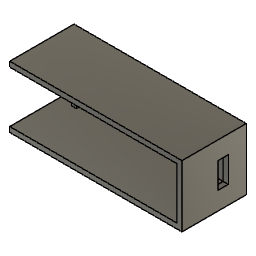
usb-bracket v4 (Autodesk Fusion 360 design; units mm, degrees)
Autodesk Fusion 360 part; units mm, degrees
sketch "Sketch1" plane through (0, 0, 0) normal (0, 1, 0) x (1, 0, 0)
  line L0 (0, 0) -> (-58, 0)
  line L1 (-58, 0) -> (-58, -20)
  line L2 (-58, -20) -> (0, -20)
  line L3 (0, -20) -> (0, 0)
  constraint horizontal L0
  constraint vertical L1
  constraint horizontal L2
  constraint vertical L3
  constraint coincident L0.start L3.end
extrude "Extrude1" add sketch "Sketch1" against normal blind 2
sketch "Sketch2" plane through (0, 0, 0) normal (0, 1, 0) x (1, 0, 0)
  line L0 (-60, -22) -> (2, -22)
  line L1 (2, -22) -> (2, -20)
  line L2 (2, -20) -> (-60, -20)
  line L3 (-60, -20) -> (-60, -22)
  constraint horizontal L0
  constraint vertical L1
  constraint horizontal L2
  constraint vertical L3
extrude "Extrude2" add sketch "Sketch2" against normal blind 7
sketch "Sketch3" plane through (0, 0, 0) normal (0, 1, 0) x (1, 0, 0)
  line L0 (-60, 0) -> (2, 0)
  line L1 (2, 0) -> (2, 2)
  line L2 (2, 2) -> (-60, 2)
  line L3 (-60, 2) -> (-60, 0)
  constraint horizontal L0
  constraint vertical L1
  constraint horizontal L2
  constraint vertical L3
extrude "Extrude3" add sketch "Sketch3" against normal blind 7
sketch "Sketch4" plane through (0, 0, 0) normal (0, 1, 0) x (1, 0, 0)
  line L0 (0, -20) -> (2, -20)
  line L1 (2, -20) -> (2, 0)
  line L2 (2, 0) -> (0, 0)
  line L3 (0, 0) -> (0, -20)
  constraint horizontal L0
  constraint vertical L1
  constraint horizontal L2
  constraint vertical L3
extrude "Extrude4" add sketch "Sketch4" against normal blind 7
sketch "Sketch5" plane through (0, 0, 0) normal (0, 1, 0) x (1, 0, 0)
  line L0 (-42, -20) -> (-37, -20)
  line L1 (-37, -20) -> (-37, 0)
  line L2 (-37, 0) -> (-42, 0)
  line L3 (-42, 0) -> (-42, -20)
  constraint horizontal L0
  constraint vertical L1
  constraint horizontal L2
  constraint vertical L3
sketch "Sketch6" plane through (0, 0, 0) normal (0, 1, 0) x (1, 0, 0)
extrude "Extrude5" add sketch "Sketch5" against normal blind 5
sketch "Sketch7" plane through (0, 0, 0) normal (0, 1, 0) x (1, 0, 0)
  line L0 (-15, -20) -> (-20, -20)
  line L1 (-20, -20) -> (-20, 0)
  line L2 (-20, 0) -> (-15, 0)
  line L3 (-15, 0) -> (-15, -20)
  constraint horizontal L0
  constraint vertical L1
  constraint horizontal L2
  constraint vertical L3
extrude "Extrude6" add sketch "Sketch7" against normal blind 5
extrude "Extrude7" add 1 faces at (-60, -2.3333, 20.6667) along direction (-1, 0, 0) blind 5
extrude "Extrude8" add 1 faces at (-60, -2.3333, -1.3333) along direction (-1, 0, 0) blind 5
extrude "Extrude9" add 1 faces at (-21, -7, -1.3333) along direction (0, -1, 0) blind 18
sketch "Sketch8" plane through (0, 0, 0) normal (1, 0, 0) x (0, 1, 0)
  line L0 (-7, 5) -> (-11, 5)
  line L1 (-11, 5) -> (-11, 15)
  line L2 (-11, 15) -> (-7, 15)
  line L3 (-7, 15) -> (-7, 5)
  constraint horizontal L0
  constraint vertical L1
  constraint horizontal L2
  constraint vertical L3
extrude "Extrude10" cut sketch "Sketch8" along normal blind 2
sketch "Sketch9" plane through (0, 0, 0) normal (0, 1, 0) x (1, 0, 0)
  line L0 (-60, -20) -> (-58, -20)
  line L1 (-58, -20) -> (-58, 0)
  line L2 (-58, 0) -> (-60, 0)
  line L3 (-60, 0) -> (-60, -20)
  dimension "d21" = 2
  constraint horizontal L0
  constraint vertical L1
  constraint horizontal L2
  constraint vertical L3
  measures "d21" distance of L0.start L0.end
extrude "Extrude11" add sketch "Sketch9" against normal blind 6
